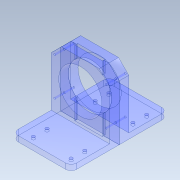
# Autodesk Inventor part: back_motor_fix_board
Saved by Autodesk Inventor 2020 (Build 240168000, 168)
## iProperties
Created: 2021-02-01
Part Number: back_motor_fix_board
Material: Generic
Document SubType Name: Modeling
Designer: DELL
Density: 1 g/cm^3
Appearance: Clear - Blue
Author: DELL
Autodesk Inventor part; units mm, degrees
ref_plane "YZ Plane" through (0, 0, 0) normal (1, 0, 0) x (0, 1, 0)
ref_plane "XZ Plane" through (0, 0, 0) normal (0, 1, 0) x (-1, 0, 0)
ref_plane "XY Plane" through (0, 0, 0) normal (0, 0, 1) x (1, 0, 0)
sketch "Sketch1" plane through (0, 0, 0) normal (0, 1, 0) x (-1, 0, 0)
  line L0 (42.5, -70) -> (-42.5, -70)
  line L1 (-42.5, -70) -> (-42.5, 70)
  line L2 (-42.5, 70) -> (42.5, 70)
  line L3 (42.5, 70) -> (42.5, -70)
  line L4 (42.5, -70) -> (-42.5, 70) construction
  line L5 (-42.5, -70) -> (42.5, 70) construction
  line L6 (-27.5, 55) -> (27.5, 55) construction
  line L7 (27.5, 55) -> (27.5, -55) construction
  line L8 (27.5, -55) -> (-27.5, -55) construction
  line L9 (-27.5, -55) -> (-27.5, 55) construction
  line L10 (-27.5, 55) -> (27.5, -55) construction
  line L11 (27.5, 55) -> (-27.5, -55) construction
  line L12 (-27.5, 35) -> (27.5, 35) construction
  line L13 (27.5, 35) -> (27.5, -35) construction
  line L14 (27.5, -35) -> (-27.5, -35) construction
  line L15 (-27.5, -35) -> (-27.5, 35) construction
  line L16 (-27.5, 35) -> (27.5, -35) construction
  line L17 (27.5, 35) -> (-27.5, -35) construction
  circle A0 centre (27.5, -55) radius 1.25
  circle A1 centre (27.5, -35) radius 1.25
  circle A2 centre (27.5, 35) radius 1.25
  circle A3 centre (27.5, 55) radius 1.25
  circle A4 centre (-27.5, -55) radius 1.25
  circle A5 centre (-27.5, -35) radius 1.25
  circle A6 centre (-27.5, 35) radius 1.25
  circle A7 centre (-27.5, 55) radius 1.25
  circle A8 centre (27.5, -55) radius 2.25
  circle A9 centre (27.5, -35) radius 2.25
  circle A10 centre (27.5, 35) radius 2.25
  circle A11 centre (27.5, 55) radius 2.25
  circle A12 centre (-27.5, 55) radius 2.25
  circle A13 centre (-27.5, 35) radius 2.25
  circle A14 centre (-27.5, -35) radius 2.25
  circle A15 centre (-27.5, -55) radius 2.25
  line L18 (-42.5, 0) -> (42.5, 0)
  point P0 (0, 0)
  dimension "d0" = 140
  dimension "d1" = 85
  dimension "d8" = 55
  dimension "d9" = 70
  dimension "d10" = 110
  dimension "d11" = 2.5
  dimension "d12" = 4.5
  constraints: 38 end point, 16 centre point, 16 coincident, 14 equal radius, 8 midpoint, 6 parallel, 3 horizontal, 3 perpendicular, 1 point on line
  measures "d0" distance of L2.end L0.start
  measures "d1" distance of L0.start L0.end
  measures "d8" distance of L6.start L6.end
  measures "d9" distance of L12.end L13.end
  measures "d10" distance between parallel lines of L6 L8
  measures "d11" diameter of A0
  measures "d12" diameter of A8
extrude "Extrusion1" add sketch "Sketch1" along normal blind 8 contours L0 L1 L18 L3 | A0 | A1 | A4 | A5 | A8 | A9 | A14 | A15
sketch "Sketch2" plane through (0, 0, 0) normal (0, 0, 1) x (1, 0, 0)
  line L0 (-42.5, 80.5) -> (-42.5, 8)
  line L1 (42.5, 80.5) -> (42.5, 8)
  line L2 (0, 0) -> (0, 53) construction
  circle A0 centre (0, 53) radius 31.5
  line L3 (-27.5, 95.5) -> (27.5, 95.5)
  line L4 (-42.5, 80.5) -> (-27.5, 95.5)
  line L5 (27.5, 95.5) -> (42.5, 80.5)
  circle A1 centre (37.5, 25.5) radius 1.25
  circle A2 centre (37.5, 80.5) radius 1.25
  circle A3 centre (37.5, 25.5) radius 2.25
  circle A4 centre (37.5, 80.5) radius 2.25
  circle A5 centre (0, 53) radius 36 construction
  line L6 (0, 53) -> (-31.1769, 71) construction
  line L7 (0, 53) -> (-31.1769, 35) construction
  line L8 (0, 53) -> (31.1769, 35) construction
  line L9 (0, 53) -> (31.1769, 71) construction
  circle A6 centre (-31.1769, 35) radius 1.65
  circle A7 centre (-31.1769, 71) radius 1.65
  circle A8 centre (0, 17) radius 1.65
  circle A9 centre (31.1769, 71) radius 1.65
  circle A10 centre (31.1769, 35) radius 1.65
  circle A11 centre (0, 89) radius 1.65
  circle A12 centre (-31.1769, 35) radius 2.75
  circle A13 centre (-31.1769, 71) radius 2.75
  circle A14 centre (0, 17) radius 2.75
  circle A15 centre (0, 89) radius 2.75
  circle A16 centre (31.1769, 35) radius 2.75
  circle A17 centre (31.1769, 71) radius 2.75
  circle A18 centre (-37.5, 25.5) radius 2.25
  circle A19 centre (-37.5, 25.5) radius 1.25
  circle A20 centre (-37.5, 80.5) radius 2.25
  circle A21 centre (-37.5, 80.5) radius 1.25
  line L10 (0, 53) -> (-36, 53) construction
  line L11 (37.5, 25.5) -> (-37.5, 80.5) construction
  line L12 (37.5, 80.5) -> (-37.5, 25.5) construction
  line L13 (-42.5, 8) -> (42.5, 8) projected
  line L14 (42.5, 8) -> (-42.5, 8)
  line L15 (42.5, 0) -> (42.5, 8) projected
  line L16 (-42.5, 0) -> (-42.5, 8) projected
  dimension "d15" = 63
  dimension "d19" = 45
  dimension "d21" = 15
  dimension "d29" = 2.5
  dimension "d30" = 55
  dimension "d31" = 4.5
  dimension "d32" = 72
  dimension "d33" = 3.3
  dimension "d34" = 5.5
  dimension "d35" = 75
  dimension "d37" = 60
  dimension "d44" = 87.5
  dimension "d45" = 45
  constraints: 28 end point, 22 centre point, 16 coincident, 16 equal radius, 5 symmetric about line, 4 point on circle, 3 collinear, 3 vertical, 3 vertical alignment, 2 horizontal, 2 horizontal alignment, 2 point on line, 1 midpoint, 1 other
  measures "d15" diameter of A0
  measures "d19" angle of L3 L4
  measures "d21" horizontal distance of L0.start L3.start
  measures "d29" diameter of A2
  measures "d30" distance of L12.start L11.start
  measures "d31" diameter of A3
  measures "d32" diameter of A5
  measures "d33" diameter of A6
  measures "d34" diameter of A16
  measures "d35" distance of A18.centre L11.start
  measures "d37" angle of L2 L8
  measures "d44" distance between parallel lines of L14 L3
  measures "d45" distance between parallel lines of L13 L10
extrude "Extrusion2" add sketch "Sketch2" against normal blind 14 contours L4 L3 L5 L1 L13 L0 | A0 | A3 | A4 | A6 | A7 | A8 | A9 | A10 | A11 | A12 | A13 | A14 | A15 | A16 | A17 | A18 | A20
extrude "Extrusion3" cut sketch "Sketch1" along normal blind 3 contours A0 | A1 | A2 | A3 | A4 | A5 | A6 | A7 | A8 | A9 | A10 | A11 | A12 | A13 | A14 | A15
extrude "Extrusion4" cut sketch "Sketch2" along normal through all both and the other way through all contours A0
sketch "Sketch4" plane through (0, 8, 0) normal (0, 1, 0) x (1, 0, 0)
  line L0 (42.5, 70) -> (-42.5, 70)
  point P0 (0, 0)
  constraints: 2 end point, 1 horizontal
sketch "Sketch3" plane through (0, 0, 0) normal (1, 0, 0) x (0, 1, 0)
  line L0 (95.5, 0) -> (95.5, -14) projected
  line L1 (95.5, -2) -> (12, -2)
  arc A0 (12, -2) -> (8, -14) centre (28, -14) ccw
  line L2 (0, 0) -> (95.5, 0) construction
  line L3 (95.5, 0) -> (95.5, -14) construction
  line L4 (95.5, -2) -> (95.5, -14)
  line L5 (8, -70) -> (8, -14) projected
  line L6 (8, -70) -> (8, -14)
  line L7 (80.5, -14) -> (8, -14) projected
  dimension "d23" = 20
  dimension "d24" = 12
  constraints: 9 end point, 2 point on circle, 2 point on line, 2 vertical, 1 centre point, 1 horizontal
  measures "d23" radius of A0
  measures "d24" distance from line of L0.end L1
surface_sweep "SweepSrf1"
split "Split1" [suppressed]
extrude "Extrusion5" [suppressed]
extrude "Extrusion6" [suppressed]
extrude "Extrusion7" [suppressed]
mirror "Mirror1" [suppressed]
mirror "Mirror2" [suppressed]
sketch "Sketch5" plane through (0, 0, 0) normal (0, -1, 0) x (1, 0, 0)
  line L0 (20, 2) -> (-20, 2)
  line L1 (-20, 2) -> (-20, -2)
  line L2 (-20, -2) -> (20, -2)
  line L3 (20, -2) -> (20, 2)
  line L4 (20, 2) -> (-20, -2) construction
  line L5 (-20, 2) -> (20, -2) construction
  point P0 (0, 0)
  dimension "d46" = 4
  dimension "d47" = 40
  constraints: 12 end point, 2 midpoint, 2 parallel, 1 horizontal, 1 perpendicular
  measures "d46" distance of L0.end L1.end
  measures "d47" distance of L0.start L0.end
extrude "Extrusion8" cut sketch "Sketch5" against normal through all
mirror "Mirror3" about plane through (0, 0, 0) normal (0, 0, 1) separate body
fillet "Fillet1" radius 8 4 edges at (-42.5, 4, -70) (42.5, 4, -70) (42.5, 4, 70) (-42.5, 4, 70)
body "Solid1"
body "Srf1"
body "Solid6"
body "Solid7"
body "Solid2"
body "Solid3"
